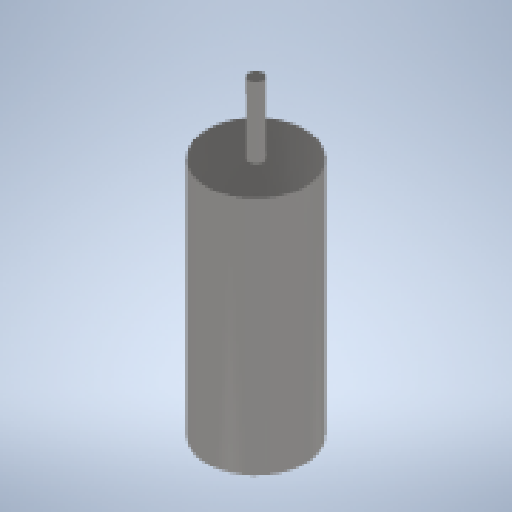
# Autodesk Inventor part: motor
Saved by Autodesk Inventor 2023.1 (Build 271208000, 208)
## iProperties
Created: 2023-05-03
Part Number: motor
Material: Steel
Document SubType Name: Modeling
Designer: felip
Density: 7.85 g/cm^3
Appearance: Steel - Polished
Author: felip
Autodesk Inventor part; units mm, degrees
ref_plane "YZ Plane" through (0, 0, 0) normal (1, 0, 0) x (0, 1, 0)
ref_plane "XZ Plane" through (0, 0, 0) normal (0, 1, 0) x (-1, 0, 0)
ref_plane "XY Plane" through (0, 0, 0) normal (0, 0, 1) x (1, 0, 0)
sketch "Sketch1" plane through (0, 0, 0) normal (0, 1, 0) x (-1, 0, 0)
  circle A0 centre (0, 0) radius 3.5
  dimension "d0" = 7
  constraints: 1 centre point, 1 coincident
  measures "d0" diameter of A0
extrude "Extrusion1" add sketch "Sketch1" along normal blind 17
sketch "Sketch2" plane through (0, 17, 0) normal (0, 1, 0) x (1, 0, 0)
  circle A0 centre (0, 0) radius 0.5
  dimension "d3" = 1
  constraints: 1 centre point, 1 coincident
  measures "d3" diameter of A0
extrude "Extrusion2" add sketch "Sketch2" along normal blind 5
sketch "Sketch3" plane through (0, 22, 0) normal (0, 1, 0) x (1, 0, 0)
  circle A0 centre (0, 0) radius 0.5 projected
  line L0 (-0.0995, 0.49) -> (0.0995, 0.49)
  circle A1 centre (0, 0) radius 0.5 projected
  line L1 (0.4999, 0.0075) -> (0.4999, 0.0075)
  line L2 (0.49, 0.0995) -> (0.49, -0.0995)
  dimension "d8" = 0.49
  dimension "d9" = 0.49
  constraints: 6 end point, 6 point on circle, 1 horizontal, 1 tangent, 1 vertical
  measures "d8" distance from line of point (0, 0) L2
  measures "d9" distance from line of L0 point (0, 0)
extrude "Extrusion3" cut sketch "Sketch3" against normal blind 0.1 contours A0 L2 | L0 A0
body "Solid1"
